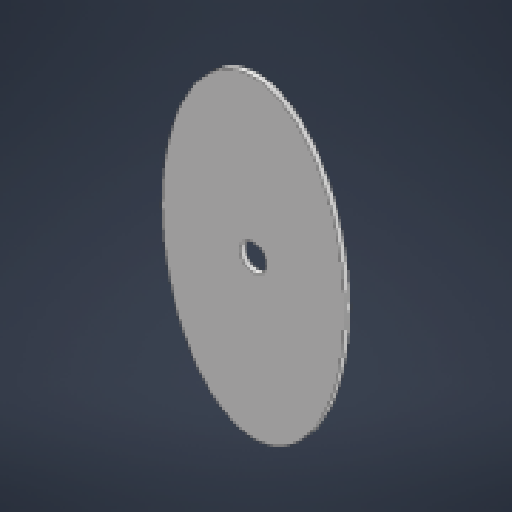
# Autodesk Inventor part: верхний эллипс туловища
Saved by Autodesk Inventor 2023.2 (Build 272271030, 271C)
## iProperties
Created: 2024-11-21
Part Number: верхний эллипс туловища
Material: Типовые
Document SubType Name: Modeling
Designer: DELL
Density: 1 g/cm^3
Appearance: По умолчанию
Author: DELL
Autodesk Inventor part; units mm, degrees
ref_plane "YZ Plane" through (0, 0, 0) normal (1, 0, 0) x (0, 1, 0)
ref_plane "XZ Plane" through (0, 0, 0) normal (0, 1, 0) x (-1, 0, 0)
ref_plane "XY Plane" through (0, 0, 0) normal (0, 0, 1) x (1, 0, 0)
sketch "Эскиз1" plane through (0, 0, 0) normal (0, 0, 1) x (1, 0, 0)
  ellipse E0 centre (0, 0) end of major axis (0.8348, -119.9971) minor radius 70
  circle A0 centre (0, 0) radius 10
  line L0 (-1.5357, -9.8814) -> (-1.5357, 9.8814)
  point P0 (-2.6143, 119.9459)
  dimension "d0" = 120
  dimension "d1" = 70
  dimension "d4" = 20
  constraints: 2 coincident, 2 end point, 2 point on circle, 1 centre point, 3 other
  measures "d4" diameter of A0
extrude "Выдавливание1" add sketch "Эскиз1" against normal blind 4
sketch "Эскиз4" plane through (0, 0, 0) normal (0, 0, 1) x (1, 0, 0)
  ellipse E0 centre (0, 0) end of major axis (0.8348, -119.9971) minor radius 70 construction
  circle A0 centre (0, 0) radius 10 construction
  ellipse E1 centre (0, 0) end of major axis (0.8348, -119.9971) minor radius 70 projected
  line L0 (0, 119.9944) -> (0, -119.9944)
  line L1 (-27.5485, 78.2738) -> (-23.5485, 78.2738)
  line L2 (-23.5485, 78.2738) -> (-23.5485, 48.2738)
  line L3 (-23.5485, 48.2738) -> (-27.5485, 48.2738)
  line L4 (-27.5485, 48.2738) -> (-27.5485, 78.2738)
  dimension "d16" = 4
  dimension "d17" = 30
  constraints: 10 end point, 2 parallel, 1 horizontal, 1 perpendicular, 1 vertical, 3 other
  measures "d16" distance of L2.end L3.end
  measures "d17" distance of L1.end L2.end
